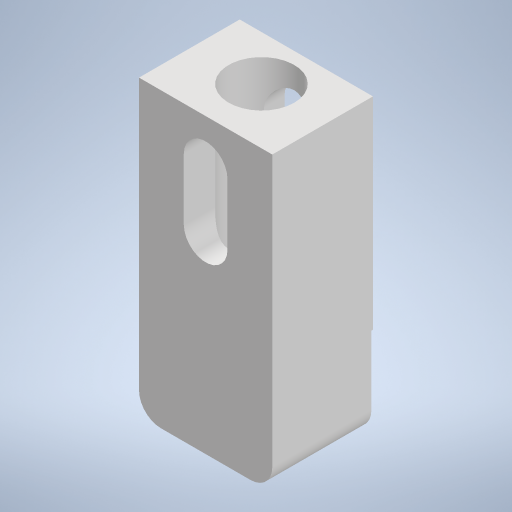
# Autodesk Inventor part: reinforced_holder
Saved by Autodesk Inventor 2024 (Build 280153000, 153)
## iProperties
Created: 2023-05-03
Part Number: reinforced_holder
Material: Generic
Document SubType Name: Modeling
Designer: Rober
Mass: 538.313 g
Surface Area: 676.575 cm^2
Volume: 538.313 cm^3
Density: 1 g/cm^3
Appearance: Default
Author: Rober
Autodesk Inventor part; units mm, degrees
ref_plane "YZ Plane" through (0, 0, 0) normal (1, 0, 0) x (0, 1, 0)
ref_plane "XZ Plane" through (0, 0, 0) normal (0, 1, 0) x (-1, 0, 0)
ref_plane "XY Plane" through (0, 0, 0) normal (0, 0, 1) x (1, 0, 0)
sketch "Sketch1" plane through (0, 0, 0) normal (0, 1, 0) x (-1, 0, 0)
  line L0 (3.05, -5.3255) -> (-3.05, -5.3255)
  line L1 (-3.05, -5.3255) -> (-3.05, 4.8245)
  line L2 (-3.05, 4.8245) -> (3.05, 4.8245)
  line L3 (3.05, 4.8245) -> (3.05, -5.3255)
  line L4 (0.9, 4.8245) -> (-0.9, 4.8245)
  line L5 (0.9, 4.8245) -> (0.9, -5.3255)
  line L6 (-0.9, 4.8245) -> (-0.9, -5.3255)
  circle A0 centre (0, 3.486) radius 0.8
  circle A1 centre (-0.0087, -3.8255) radius 0.8
  line L7 (0, 4.8245) -> (0, -5.3255)
  line L8 (-3.05, 0) -> (3.05, 0)
  point P0 (0, 0)
  dimension "d13" = 6.1
  dimension "d44" = 1.8
  dimension "d45" = 2.15
  dimension "d46" = 1.6
  dimension "d47" = 1.6
  constraints: 18 end point, 8 point on line, 4 perpendicular, 3 midpoint, 2 centre point, 2 parallel, 1 horizontal
  measures "d13" distance of L0.start L0.end
  measures "d44" distance of L4.start L4.end
  measures "d45" distance from line of L3 L4.start
  measures "d46" diameter of A0
  measures "d47" diameter of A1
extrude "Extrusion1" add sketch "Sketch1" along normal blind 10.15 contours L0 L5 L8 L3 | L0 L7 A1 L8 L5 | L8 L5 L2 L3 | L0 L6 L8 L7 A1 | L8 L7 A0 L2 L5 | L0 L1 L8 L6 | L8 L6 L2 L7 A0 | L8 L1 L2 L6
sketch "Sketch11" plane through (-3.05, 0, 4.8245) normal (0, 0, 1) x (1, 0, 0)
  point P0 (3.05, 0)
extrude "Extrusion6" add sketch "Sketch1" against normal blind 1 contours L0 L7 A1 L8 L5 | L0 L6 L8 L7 A1 | L8 L7 A0 L2 L5 | L8 L6 L2 L7 A0
sketch "Sketch12" plane through (0, 10.15, 0) normal (0, 1, 0) x (1, 0, 0)
  circle A0 centre (0.0087, 3.8255) radius 1.265
  circle A1 centre (0, -3.486) radius 1.265
  circle A2 centre (0, -3.486) radius 0.8 projected
  circle A3 centre (0.0087, 3.8255) radius 0.8 projected
  point P0 (0, 0)
  dimension "d52" = 2.53
  dimension "d53" = 2.53
  constraints: 2 centre point, 2 concentric
  measures "d52" diameter of A0
  measures "d53" diameter of A1
extrude "Extrusion7" cut sketch "Sketch12" against normal blind 1 contours A0 | A1 | A2 | A3
sketch "Sketch13" plane through (-3.05, 10.15, 4.8245) normal (0, 0, 1) x (1, 0, 0)
  line L0 (0, 0) -> (0, -4.15)
  line L1 (0, -10.15) -> (0, 0) projected
  line L2 (0, -4.15) -> (6.1, -4.15)
  line L3 (6.1, -10.15) -> (6.1, 0) projected
  line L4 (6.1, 0) -> (6.1, -4.15)
  line L5 (0, 0) -> (6.1, 0)
  point P0 (3.05, -10.15)
  dimension "d56" = 4.15
  constraints: 8 end point, 3 perpendicular, 2 point on line
  measures "d56" distance of L0.start L0.end
extrude "Extrusion8" add sketch "Sketch13" along normal blind 17
sketch "Sketch17" plane through (-3.05, 10.15, 21.8245) normal (0, 0, 1) x (1, 0, 0)
  line L0 (6.1, 0) -> (0, 0) projected
  line L1 (6.1, 0) -> (14.3904, 5.5919)
  line L2 (6.1, 0) -> (16.1, 0) construction
  line L3 (14.3904, 5.5919) -> (10.1964, 11.8097)
  line L4 (10.1964, 11.8097) -> (13.5955, 14.1024)
  line L5 (13.5955, 14.1024) -> (17.7894, 7.8846)
  line L6 (17.7894, 7.8846) -> (19.7132, 5.0325)
  line L7 (6.1, -10.15) -> (6.1, -4.15) projected
  line L8 (19.7132, 5.0325) -> (6.1, -4.15)
  line L9 (6.1, 0) -> (6.1, -4.15)
  point P0 (3.05, -10.15)
  dimension "d72" = 10
  dimension "d73" = 34
  dimension "d74" = 7.5
  dimension "d75" = 4.1
  constraints: 16 end point, 3 perpendicular, 2 point on line, 1 equal length, 1 horizontal, 1 vertical
  measures "d72" distance of L0.start L1.end
  measures "d73" angle of L2 L1
  measures "d74" distance of L1.end L3.end
  measures "d75" distance of L3.end L4.end
extrude "Extrusion12" [suppressed]
sketch "Sketch14" plane through (0, 10.15, 0) normal (0, 1, 0) x (1, 0, 0)
  line L0 (3.05, 5.3255) -> (3.05, -21.8245) projected
  line L1 (3.05, -21.8245) -> (3.05, -17.7145)
  line L2 (3.05, -17.7145) -> (-3.05, -17.7145)
  line L3 (-3.05, 5.3255) -> (-3.05, -21.8245) projected
  line L4 (-3.05, -21.8245) -> (3.05, -21.8245)
  point P0 (0, 0)
  dimension "d59" = 4.11
  constraints: 6 end point, 2 point on line, 1 parallel, 1 perpendicular
  measures "d59" distance of L0.end L1.end
extrude "Extrusion9" add sketch "Sketch14" along normal blind 9.25
sketch "Sketch16" plane through (0, 19.4, 0) normal (0, 1, 0) x (1, 0, 0)
  circle A0 centre (0, -19.7695) radius 1.5
  line L0 (-3.05, -21.8245) -> (3.05, -21.8245) projected
  line L1 (3.05, -21.8245) -> (3.05, -17.7145) projected
  point P0 (0, 0)
  point P1 (0, -21.8245)
  dimension "d67" = 3
  dimension "d68" = 2.055
  dimension "d69" = 3.05
  constraints: 1 centre point, 1 midpoint
  measures "d67" diameter of A0
  measures "d68" distance of point (0, -21.824) A0.centre
  measures "d69" distance from line of L1 A0.centre
extrude "Extrusion11" cut sketch "Sketch16" against normal blind 10
sketch "Sketch15" plane through (-3.05, 10.15, 21.8245) normal (0, 0, 1) x (1, 0, 0)
  line L0 (3.05, 7.25) -> (3.05, 4.45) construction
  line L1 (6.1, 0) -> (6.1, 9.25) projected
  line L2 (2.05, 7.25) -> (2.05, 4.45)
  line L3 (4.05, 4.45) -> (4.05, 7.25)
  arc A0 (4.05, 7.25) -> (2.05, 7.25) centre (3.05, 7.25) ccw
  arc A1 (2.05, 4.45) -> (4.05, 4.45) centre (3.05, 4.45) ccw
  line L4 (0, 9.25) -> (6.1, 9.25) projected
  line L5 (3.05, 9.25) -> (3.05, 8.25)
  point P0 (3.05, -10.15)
  point P1 (3.05, 5.85)
  dimension "d62" = 1.4
  dimension "d63" = 2
  dimension "d64" = 3.05
  dimension "d94" = 2.05
  dimension "d97" = 1
  constraints: 10 end point, 5 point on circle, 4 tangent, 2 centre point, 2 midpoint, 2 parallel
  measures "d62" distance of point (3.05, 5.85) L0.end
  measures "d63" diameter of A1
  measures "d64" distance from line of L1 point (3.05, 5.85)
  measures "d94" distance between parallel lines of L3 L1
  measures "d97" distance of L5.start L5.end
extrude "Extrusion10" cut sketch "Sketch15" against normal through all
sketch "Sketch20" plane through (10.5455, 24.2524, 21.8245) normal (-0.5591929, 0.8290376, 0) x (0.8290376, 0.5591929, 0)
  circle A0 centre (-2.05, 2.05) radius 1.5
  line L0 (-4.1, 0) -> (-4.1, 4.1) projected
  line L1 (0, 0) -> (-4.1, 0) projected
  point P0 (-22.3044, 21.8245)
  point P1 (-2.05, 0)
  dimension "d82" = 3
  dimension "d83" = 2.05
  dimension "d84" = 2.05
  constraints: 1 centre point, 1 midpoint
  measures "d82" diameter of A0
  measures "d83" distance from line of L0 A0.centre
  measures "d84" distance of point (-2.05, 0) A0.centre
extrude "Extrusion14" [suppressed]
sketch "Sketch18" plane through (-3.05, 10.15, 21.8245) normal (0, 0, 1) x (1, 0, 0)
  line L0 (12.6984, 11.7664) -> (14.2641, 9.4451) construction
  line L1 (11.973, 11.2771) -> (13.5387, 8.9558)
  line L2 (14.9895, 9.9344) -> (13.4238, 12.2557)
  arc A0 (13.4238, 12.2557) -> (11.973, 11.2771) centre (12.6984, 11.7664) ccw
  arc A1 (13.5387, 8.9558) -> (14.9895, 9.9344) centre (14.2641, 9.4451) ccw
  line L3 (19.7132, 5.0325) -> (13.5955, 14.1024) projected
  line L4 (10.1964, 11.8097) -> (13.5955, 14.1024) projected
  point P0 (3.05, -10.15)
  point P1 (13.4813, 10.6057)
  point P2 (12.2091, 12.4918)
  dimension "d78" = 1.4
  dimension "d79" = 1.75
  dimension "d89" = 0.56
  dimension "d90" = 2.05
  constraints: 8 end point, 5 point on circle, 4 tangent, 2 centre point, 2 parallel, 1 midpoint
  measures "d78" distance of point (13.481, 10.606) L0.end
  measures "d79" diameter of A1
  measures "d89" distance from line of L4 point (12.209, 12.492)
  measures "d90" distance from line of L3 point (13.481, 10.606)
extrude "Extrusion13" cut sketch "Sketch18" against normal blind 4.1
sketch "Sketch21" plane through (13.8787, 15.6447, 19.7745) normal (-0.5591929, 0.8290376, 0) x (0.8290376, 0.5591929, 0)
  circle A0 centre (0, 0) radius 0.868
  point P0 (-20.2544, 19.7745)
  constraints: 1 centre point
extrude "Extrusion15" [suppressed]
mirror "Mirror3" about plane through (0, 0, 0) normal (1, 0, 0) of "Extrusion13"
fillet "Fillet1" radius 1 2 edges at (3.05, 10.15, 6.1945) (-3.05, 10.15, 6.1945)
fillet "Fillet2" [suppressed]
fillet "Fillet3" radius 1 2 edges at (3.05, 6, 13.3245) (-3.05, 6, 13.3245)
sketch "Sketch33" plane through (-3.05, 10.15, 21.8245) normal (0, 0, 1) x (1, 0, 0)
  line L0 (4.05, 7.25) -> (4.05, 4.45) projected
  arc A0 (2.05, 4.45) -> (4.05, 4.45) centre (3.05, 4.45) ccw projected
  line L1 (2.05, 4.45) -> (2.05, 7.25) projected
  arc A1 (4.05, 7.25) -> (2.05, 7.25) centre (3.05, 7.25) ccw projected
  arc A2 (0, -3.15) -> (1, -4.15) centre (1, -3.15) ccw projected
  line L2 (1, -4.15) -> (5.1, -4.15) projected
  arc A3 (5.1, -4.15) -> (6.1, -3.15) centre (5.1, -3.15) ccw projected
  line L3 (6.1, -3.15) -> (6.1, 9.25) projected
  line L4 (0, 9.25) -> (6.1, 9.25) projected
  line L5 (0, -3.15) -> (0, 9.25) projected
  point P0 (3.05, -10.15)
extrude "Extrusion17" add sketch "Sketch33" along normal blind 0.5
sketch "Sketch36" plane through (0, 10.15, 0) normal (0, 1, 0) x (1, 0, 0)
  line L0 (3.05, -17.7145) -> (3.05, 5.3255) projected
  line L1 (-3.5916, 5.3255) -> (3.05, 5.3255)
  line L2 (3.05, 5.3255) -> (3.05, -17.7864)
  line L3 (3.05, -17.7864) -> (-3.5916, -17.7864)
  line L4 (-3.5916, -17.7864) -> (-3.5916, 5.3255)
  point P0 (0, 0)
  point P1 (3.05, 5.3255)
  constraints: 8 end point, 2 parallel, 1 horizontal, 1 perpendicular, 1 point on line
extrude "Extrusion18" cut sketch "Sketch36" against normal through all
sketch "Sketch22" plane through (0, 9.4, 19.7695) normal (0, 1, 0) x (1, 0, 0)
  circle A0 centre (0, 0) radius 1.5 projected
  point P0 (0, 19.7695)
extrude "Extrusion16" [suppressed]
equation "\"d13\" = base_width"
equation "\"d45\" = -0.5 * d44 + 0.5 * d13"
equation "\"d4\" = base_length"
equation "\"base_width\" = 6.1"
equation "\"base_length\" = 10.15"
equation "\"base_screw_diameter\" = 1.5"
equation "\"base_screw_spacing_edge\" = 8.5"
equation "\"multi_angle\" = 34deg"
body "Solid1"
